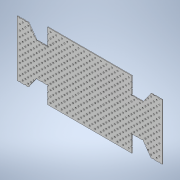
# Autodesk Inventor part: buildplate1
Saved by Autodesk Inventor 2020.1 (Build 241239000, 239)
## iProperties
Created: 2019-12-09
Part Number: buildplate1
Material: Aluminum 6061
Document SubType Name: Modeling
Designer: tbloo
Density: 2.7 g/cm^3
Appearance: Aluminum - Dark
Author: tbloo
Autodesk Inventor part; units mm, degrees
(part 1 of 2)
ref_plane "YZ Plane" through (0, 0, 0) normal (1, 0, 0) x (0, 1, 0)
ref_plane "XZ Plane" through (0, 0, 0) normal (0, 1, 0) x (-1, 0, 0)
ref_plane "XY Plane" through (0, 0, 0) normal (0, 0, 1) x (1, 0, 0)
sketch "Sketch1" plane through (0, 0, 0) normal (0, 0, 1) x (1, 0, 0)
  point P0 (0, 0)
sketch "Sketch2" plane through (0, 0, 0) normal (0, 0, 1) x (1, 0, 0)
  line L0 (32, 144) -> (-384, 144)
  line L1 (-384, 144) -> (-384, -48)
  line L2 (-384, -48) -> (32, -48)
  line L3 (32, -48) -> (32, 144)
  circle A0 centre (24, 128) radius 1.85
  circle A1 centre (16, 136) radius 1.85
  circle A2 centre (24, 112) radius 1.85
  circle A3 centre (16, 120) radius 1.85
  circle A4 centre (8, 128) radius 1.85
  circle A5 centre (0, 136) radius 1.85
  circle A6 centre (24, 112) radius 1.85
  circle A7 centre (16, 120) radius 1.85
  circle A8 centre (8, 112) radius 1.85
  circle A9 centre (16, 104) radius 1.85
  circle A10 centre (24, 96) radius 1.85
  circle A11 centre (16, 104) radius 1.85
  circle A12 centre (8, 96) radius 1.85
  circle A13 centre (16, 88) radius 1.85
  circle A14 centre (24, 80) radius 1.85
  circle A15 centre (16, 88) radius 1.85
  circle A16 centre (8, 80) radius 1.85
  circle A17 centre (16, 72) radius 1.85
  circle A18 centre (24, 64) radius 1.85
  circle A19 centre (16, 72) radius 1.85
  circle A20 centre (8, 64) radius 1.85
  circle A21 centre (16, 56) radius 1.85
  circle A22 centre (24, 48) radius 1.85
  circle A23 centre (16, 56) radius 1.85
  circle A24 centre (8, 48) radius 1.85
  circle A25 centre (16, 40) radius 1.85
  circle A26 centre (24, 32) radius 1.85
  circle A27 centre (16, 40) radius 1.85
  circle A28 centre (8, 32) radius 1.85
  circle A29 centre (16, 24) radius 1.85
  circle A30 centre (24, 16) radius 1.85
  circle A31 centre (16, 24) radius 1.85
  circle A32 centre (8, 16) radius 1.85
  circle A33 centre (16, 8) radius 1.85
  circle A34 centre (24, 0) radius 1.85
  circle A35 centre (16, 8) radius 1.85
  circle A36 centre (8, 0) radius 1.85
  circle A37 centre (16, -8) radius 1.85
  circle A38 centre (24, -16) radius 1.85
  circle A39 centre (16, -8) radius 1.85
  circle A40 centre (8, -16) radius 1.85
  circle A41 centre (16, -24) radius 1.85
  circle A42 centre (24, -32) radius 1.85
  circle A43 centre (16, -24) radius 1.85
  circle A44 centre (8, -32) radius 1.85
  circle A45 centre (16, -40) radius 1.85
  circle A46 centre (8, 128) radius 1.85
  circle A47 centre (0, 136) radius 1.85
  circle A48 centre (-8, 128) radius 1.85
  circle A49 centre (0, 120) radius 1.85
  circle A50 centre (8, 112) radius 1.85
  circle A51 centre (0, 120) radius 1.85
  circle A52 centre (-8, 112) radius 1.85
  circle A53 centre (0, 104) radius 1.85
  circle A54 centre (8, 96) radius 1.85
  circle A55 centre (0, 104) radius 1.85
  circle A56 centre (-8, 96) radius 1.85
  circle A57 centre (0, 88) radius 1.85
  circle A58 centre (8, 80) radius 1.85
  circle A59 centre (0, 88) radius 1.85
  circle A60 centre (-8, 80) radius 1.85
  circle A61 centre (0, 72) radius 1.85
  circle A62 centre (8, 64) radius 1.85
  circle A63 centre (0, 72) radius 1.85
  circle A64 centre (-8, 64) radius 1.85
  circle A65 centre (0, 56) radius 1.85
  circle A66 centre (8, 48) radius 1.85
  circle A67 centre (0, 56) radius 1.85
  circle A68 centre (-8, 48) radius 1.85
  circle A69 centre (0, 40) radius 1.85
  circle A70 centre (8, 32) radius 1.85
  circle A71 centre (0, 40) radius 1.85
  circle A72 centre (-8, 32) radius 1.85
  circle A73 centre (0, 24) radius 1.85
  circle A74 centre (8, 16) radius 1.85
  circle A75 centre (0, 24) radius 1.85
  circle A76 centre (-8, 16) radius 1.85
  circle A77 centre (0, 8) radius 1.85
  circle A78 centre (8, 0) radius 1.85
  circle A79 centre (0, 8) radius 1.85
  circle A80 centre (-8, 0) radius 1.85
  circle A81 centre (0, -8) radius 1.85
  circle A82 centre (8, -16) radius 1.85
  circle A83 centre (0, -8) radius 1.85
  circle A84 centre (-8, -16) radius 1.85
  circle A85 centre (0, -24) radius 1.85
  circle A86 centre (8, -32) radius 1.85
  circle A87 centre (0, -24) radius 1.85
  circle A88 centre (-8, -32) radius 1.85
  circle A89 centre (0, -40) radius 1.85
  circle A90 centre (-8, 128) radius 1.85
  circle A91 centre (-16, 136) radius 1.85
  circle A92 centre (-24, 128) radius 1.85
  circle A93 centre (-16, 120) radius 1.85
  circle A94 centre (-8, 112) radius 1.85
  circle A95 centre (-16, 120) radius 1.85
  circle A96 centre (-24, 112) radius 1.85
  circle A97 centre (-16, 104) radius 1.85
  circle A98 centre (-8, 96) radius 1.85
  circle A99 centre (-16, 104) radius 1.85
  circle A100 centre (-24, 96) radius 1.85
  circle A101 centre (-16, 88) radius 1.85
  circle A102 centre (-8, 80) radius 1.85
  circle A103 centre (-16, 88) radius 1.85
  circle A104 centre (-24, 80) radius 1.85
  circle A105 centre (-16, 72) radius 1.85
  circle A106 centre (-8, 64) radius 1.85
  circle A107 centre (-16, 72) radius 1.85
  circle A108 centre (-24, 64) radius 1.85
  circle A109 centre (-16, 56) radius 1.85
  circle A110 centre (-8, 48) radius 1.85
  circle A111 centre (-16, 56) radius 1.85
  circle A112 centre (-24, 48) radius 1.85
  circle A113 centre (-16, 40) radius 1.85
  circle A114 centre (-8, 32) radius 1.85
  circle A115 centre (-16, 40) radius 1.85
  circle A116 centre (-24, 32) radius 1.85
  circle A117 centre (-16, 24) radius 1.85
  circle A118 centre (-8, 16) radius 1.85
  circle A119 centre (-16, 24) radius 1.85
  circle A120 centre (-24, 16) radius 1.85
  circle A121 centre (-16, 8) radius 1.85
  circle A122 centre (-8, 0) radius 1.85
  circle A123 centre (-16, 8) radius 1.85
  circle A124 centre (-24, 0) radius 1.85
  circle A125 centre (-16, -8) radius 1.85
  circle A126 centre (-8, -16) radius 1.85
  circle A127 centre (-16, -8) radius 1.85
  circle A128 centre (-24, -16) radius 1.85
  circle A129 centre (-16, -24) radius 1.85
  circle A130 centre (-8, -32) radius 1.85
  circle A131 centre (-16, -24) radius 1.85
  circle A132 centre (-24, -32) radius 1.85
  circle A133 centre (-16, -40) radius 1.85
  circle A134 centre (-24, 128) radius 1.85
  circle A135 centre (-32, 136) radius 1.85
  circle A136 centre (-40, 128) radius 1.85
  circle A137 centre (-32, 120) radius 1.85
  circle A138 centre (-24, 112) radius 1.85
  circle A139 centre (-32, 120) radius 1.85
  circle A140 centre (-40, 112) radius 1.85
  circle A141 centre (-32, 104) radius 1.85
  circle A142 centre (-24, 96) radius 1.85
  circle A143 centre (-32, 104) radius 1.85
  circle A144 centre (-40, 96) radius 1.85
  circle A145 centre (-32, 88) radius 1.85
  circle A146 centre (-24, 80) radius 1.85
  circle A147 centre (-32, 88) radius 1.85
  circle A148 centre (-40, 80) radius 1.85
  circle A149 centre (-32, 72) radius 1.85
  circle A150 centre (-24, 64) radius 1.85
  circle A151 centre (-32, 72) radius 1.85
  circle A152 centre (-40, 64) radius 1.85
  circle A153 centre (-32, 56) radius 1.85
  circle A154 centre (-24, 48) radius 1.85
  circle A155 centre (-32, 56) radius 1.85
  circle A156 centre (-40, 48) radius 1.85
  circle A157 centre (-32, 40) radius 1.85
  circle A158 centre (-24, 32) radius 1.85
  circle A159 centre (-32, 40) radius 1.85
  circle A160 centre (-40, 32) radius 1.85
  circle A161 centre (-32, 24) radius 1.85
  circle A162 centre (-24, 16) radius 1.85
  circle A163 centre (-32, 24) radius 1.85
  circle A164 centre (-40, 16) radius 1.85
  circle A165 centre (-32, 8) radius 1.85
  circle A166 centre (-24, 0) radius 1.85
  circle A167 centre (-32, 8) radius 1.85
  circle A168 centre (-40, 0) radius 1.85
  circle A169 centre (-32, -8) radius 1.85
  circle A170 centre (-24, -16) radius 1.85
  circle A171 centre (-32, -8) radius 1.85
  circle A172 centre (-40, -16) radius 1.85
  circle A173 centre (-32, -24) radius 1.85
  circle A174 centre (-24, -32) radius 1.85
  circle A175 centre (-32, -24) radius 1.85
  circle A176 centre (-40, -32) radius 1.85
  circle A177 centre (-32, -40) radius 1.85
  circle A178 centre (-40, 128) radius 1.85
  circle A179 centre (-48, 136) radius 1.85
  circle A180 centre (-56, 128) radius 1.85
  circle A181 centre (-48, 120) radius 1.85
  circle A182 centre (-40, 112) radius 1.85
  circle A183 centre (-48, 120) radius 1.85
  circle A184 centre (-56, 112) radius 1.85
  circle A185 centre (-48, 104) radius 1.85
  circle A186 centre (-40, 96) radius 1.85
  circle A187 centre (-48, 104) radius 1.85
  circle A188 centre (-56, 96) radius 1.85
  circle A189 centre (-48, 88) radius 1.85
  circle A190 centre (-40, 80) radius 1.85
  circle A191 centre (-48, 88) radius 1.85
  circle A192 centre (-56, 80) radius 1.85
  circle A193 centre (-48, 72) radius 1.85
  circle A194 centre (-40, 64) radius 1.85
  circle A195 centre (-48, 72) radius 1.85
  circle A196 centre (-56, 64) radius 1.85
  circle A197 centre (-48, 56) radius 1.85
  circle A198 centre (-40, 48) radius 1.85
  circle A199 centre (-48, 56) radius 1.85
  circle A200 centre (-56, 48) radius 1.85
  circle A201 centre (-48, 40) radius 1.85
  circle A202 centre (-40, 32) radius 1.85
  circle A203 centre (-48, 40) radius 1.85
  circle A204 centre (-56, 32) radius 1.85
  circle A205 centre (-48, 24) radius 1.85
  circle A206 centre (-40, 16) radius 1.85
  circle A207 centre (-48, 24) radius 1.85
  circle A208 centre (-56, 16) radius 1.85
  circle A209 centre (-48, 8) radius 1.85
  circle A210 centre (-40, 0) radius 1.85
  circle A211 centre (-48, 8) radius 1.85
  circle A212 centre (-56, 0) radius 1.85
  circle A213 centre (-48, -8) radius 1.85
  circle A214 centre (-40, -16) radius 1.85
  circle A215 centre (-48, -8) radius 1.85
  circle A216 centre (-56, -16) radius 1.85
  circle A217 centre (-48, -24) radius 1.85
  circle A218 centre (-40, -32) radius 1.85
  circle A219 centre (-48, -24) radius 1.85
  circle A220 centre (-56, -32) radius 1.85
  circle A221 centre (-48, -40) radius 1.85
  circle A222 centre (-56, 128) radius 1.85
  circle A223 centre (-64, 136) radius 1.85
  circle A224 centre (-72, 128) radius 1.85
  circle A225 centre (-64, 120) radius 1.85
  circle A226 centre (-56, 112) radius 1.85
  circle A227 centre (-64, 120) radius 1.85
  circle A228 centre (-72, 112) radius 1.85
  circle A229 centre (-64, 104) radius 1.85
  circle A230 centre (-56, 96) radius 1.85
  circle A231 centre (-64, 104) radius 1.85
  circle A232 centre (-72, 96) radius 1.85
  circle A233 centre (-64, 88) radius 1.85
  circle A234 centre (-56, 80) radius 1.85
  circle A235 centre (-64, 88) radius 1.85
  circle A236 centre (-72, 80) radius 1.85
  circle A237 centre (-64, 72) radius 1.85
  circle A238 centre (-56, 64) radius 1.85
  circle A239 centre (-64, 72) radius 1.85
  circle A240 centre (-72, 64) radius 1.85
  circle A241 centre (-64, 56) radius 1.85
  circle A242 centre (-56, 48) radius 1.85
  circle A243 centre (-64, 56) radius 1.85
  circle A244 centre (-72, 48) radius 1.85
  circle A245 centre (-64, 40) radius 1.85
  circle A246 centre (-56, 32) radius 1.85
  circle A247 centre (-64, 40) radius 1.85
  circle A248 centre (-72, 32) radius 1.85
  circle A249 centre (-64, 24) radius 1.85
  circle A250 centre (-56, 16) radius 1.85
  circle A251 centre (-64, 24) radius 1.85
  circle A252 centre (-72, 16) radius 1.85
  circle A253 centre (-64, 8) radius 1.85
  circle A254 centre (-56, 0) radius 1.85
  circle A255 centre (-64, 8) radius 1.85
  circle A256 centre (-72, 0) radius 1.85
  circle A257 centre (-64, -8) radius 1.85
  circle A258 centre (-56, -16) radius 1.85
  circle A259 centre (-64, -8) radius 1.85
  circle A260 centre (-72, -16) radius 1.85
  circle A261 centre (-64, -24) radius 1.85
  circle A262 centre (-56, -32) radius 1.85
  circle A263 centre (-64, -24) radius 1.85
  circle A264 centre (-72, -32) radius 1.85
  circle A265 centre (-64, -40) radius 1.85
  circle A266 centre (-72, 128) radius 1.85
  circle A267 centre (-80, 136) radius 1.85
  circle A268 centre (-88, 128) radius 1.85
  circle A269 centre (-80, 120) radius 1.85
  circle A270 centre (-72, 112) radius 1.85
  circle A271 centre (-80, 120) radius 1.85
  circle A272 centre (-88, 112) radius 1.85
  circle A273 centre (-80, 104) radius 1.85
  circle A274 centre (-72, 96) radius 1.85
  circle A275 centre (-80, 104) radius 1.85
  circle A276 centre (-88, 96) radius 1.85
  circle A277 centre (-80, 88) radius 1.85
  circle A278 centre (-72, 80) radius 1.85
  circle A279 centre (-80, 88) radius 1.85
  circle A280 centre (-88, 80) radius 1.85
  circle A281 centre (-80, 72) radius 1.85
  circle A282 centre (-72, 64) radius 1.85
  circle A283 centre (-80, 72) radius 1.85
  circle A284 centre (-88, 64) radius 1.85
  circle A285 centre (-80, 56) radius 1.85
  circle A286 centre (-72, 48) radius 1.85
  circle A287 centre (-80, 56) radius 1.85
  circle A288 centre (-88, 48) radius 1.85
  circle A289 centre (-80, 40) radius 1.85
  circle A290 centre (-72, 32) radius 1.85
  circle A291 centre (-80, 40) radius 1.85
  circle A292 centre (-88, 32) radius 1.85
  circle A293 centre (-80, 24) radius 1.85
  circle A294 centre (-72, 16) radius 1.85
  circle A295 centre (-80, 24) radius 1.85
  circle A296 centre (-88, 16) radius 1.85
  circle A297 centre (-80, 8) radius 1.85
  circle A298 centre (-72, 0) radius 1.85
  circle A299 centre (-80, 8) radius 1.85
  circle A300 centre (-88, 0) radius 1.85
  circle A301 centre (-80, -8) radius 1.85
  circle A302 centre (-72, -16) radius 1.85
  circle A303 centre (-80, -8) radius 1.85
  circle A304 centre (-88, -16) radius 1.85
  circle A305 centre (-80, -24) radius 1.85
  circle A306 centre (-72, -32) radius 1.85
  circle A307 centre (-80, -24) radius 1.85
  circle A308 centre (-88, -32) radius 1.85
  circle A309 centre (-80, -40) radius 1.85
  circle A310 centre (-88, 128) radius 1.85
  circle A311 centre (-96, 136) radius 1.85
  circle A312 centre (-104, 128) radius 1.85
  circle A313 centre (-96, 120) radius 1.85
  circle A314 centre (-88, 112) radius 1.85
  circle A315 centre (-96, 120) radius 1.85
  circle A316 centre (-104, 112) radius 1.85
  circle A317 centre (-96, 104) radius 1.85
  circle A318 centre (-88, 96) radius 1.85
  circle A319 centre (-96, 104) radius 1.85
  circle A320 centre (-104, 96) radius 1.85
  circle A321 centre (-96, 88) radius 1.85
  circle A322 centre (-88, 80) radius 1.85
  circle A323 centre (-96, 88) radius 1.85
  circle A324 centre (-104, 80) radius 1.85
  circle A325 centre (-96, 72) radius 1.85
  circle A326 centre (-88, 64) radius 1.85
  circle A327 centre (-96, 72) radius 1.85
  circle A328 centre (-104, 64) radius 1.85
  circle A329 centre (-96, 56) radius 1.85
  circle A330 centre (-88, 48) radius 1.85
  circle A331 centre (-96, 56) radius 1.85
  circle A332 centre (-104, 48) radius 1.85
  circle A333 centre (-96, 40) radius 1.85
  circle A334 centre (-88, 32) radius 1.85
  circle A335 centre (-96, 40) radius 1.85
  circle A336 centre (-104, 32) radius 1.85
  circle A337 centre (-96, 24) radius 1.85
  circle A338 centre (-88, 16) radius 1.85
  circle A339 centre (-96, 24) radius 1.85
  circle A340 centre (-104, 16) radius 1.85
  circle A341 centre (-96, 8) radius 1.85
  circle A342 centre (-88, 0) radius 1.85
  circle A343 centre (-96, 8) radius 1.85
  circle A344 centre (-104, 0) radius 1.85
  circle A345 centre (-96, -8) radius 1.85
  circle A346 centre (-88, -16) radius 1.85
  circle A347 centre (-96, -8) radius 1.85
  circle A348 centre (-104, -16) radius 1.85
  circle A349 centre (-96, -24) radius 1.85
  circle A350 centre (-88, -32) radius 1.85
  circle A351 centre (-96, -24) radius 1.85
  circle A352 centre (-104, -32) radius 1.85
  circle A353 centre (-96, -40) radius 1.85
  circle A354 centre (-104, 128) radius 1.85
  circle A355 centre (-112, 136) radius 1.85
  circle A356 centre (-120, 128) radius 1.85
  circle A357 centre (-112, 120) radius 1.85
  circle A358 centre (-104, 112) radius 1.85
  circle A359 centre (-112, 120) radius 1.85
  circle A360 centre (-120, 112) radius 1.85
  circle A361 centre (-112, 104) radius 1.85
  circle A362 centre (-104, 96) radius 1.85
  circle A363 centre (-112, 104) radius 1.85
  circle A364 centre (-120, 96) radius 1.85
  circle A365 centre (-112, 88) radius 1.85
  circle A366 centre (-104, 80) radius 1.85
  circle A367 centre (-112, 88) radius 1.85
  circle A368 centre (-120, 80) radius 1.85
  circle A369 centre (-112, 72) radius 1.85
  circle A370 centre (-104, 64) radius 1.85
  circle A371 centre (-112, 72) radius 1.85
  circle A372 centre (-120, 64) radius 1.85
  circle A373 centre (-112, 56) radius 1.85
  circle A374 centre (-104, 48) radius 1.85
  circle A375 centre (-112, 56) radius 1.85
  circle A376 centre (-120, 48) radius 1.85
  circle A377 centre (-112, 40) radius 1.85
  circle A378 centre (-104, 32) radius 1.85
  circle A379 centre (-112, 40) radius 1.85
  circle A380 centre (-120, 32) radius 1.85
  circle A381 centre (-112, 24) radius 1.85
  circle A382 centre (-104, 16) radius 1.85
  circle A383 centre (-112, 24) radius 1.85
  circle A384 centre (-120, 16) radius 1.85
  circle A385 centre (-112, 8) radius 1.85
  circle A386 centre (-104, 0) radius 1.85
  circle A387 centre (-112, 8) radius 1.85
  circle A388 centre (-120, 0) radius 1.85
  circle A389 centre (-112, -8) radius 1.85
  circle A390 centre (-104, -16) radius 1.85
  circle A391 centre (-112, -8) radius 1.85
  circle A392 centre (-120, -16) radius 1.85
  circle A393 centre (-112, -24) radius 1.85
  circle A394 centre (-104, -32) radius 1.85
  circle A395 centre (-112, -24) radius 1.85
  circle A396 centre (-120, -32) radius 1.85
  circle A397 centre (-112, -40) radius 1.85
  circle A398 centre (-120, 128) radius 1.85
  circle A399 centre (-128, 136) radius 1.85
  circle A400 centre (-136, 128) radius 1.85
  circle A401 centre (-128, 120) radius 1.85
  circle A402 centre (-120, 112) radius 1.85
  circle A403 centre (-128, 120) radius 1.85
  circle A404 centre (-136, 112) radius 1.85
  circle A405 centre (-128, 104) radius 1.85
  circle A406 centre (-120, 96) radius 1.85
  circle A407 centre (-128, 104) radius 1.85
  circle A408 centre (-136, 96) radius 1.85
  circle A409 centre (-128, 88) radius 1.85
  circle A410 centre (-120, 80) radius 1.85
  circle A411 centre (-128, 88) radius 1.85
  circle A412 centre (-136, 80) radius 1.85
  circle A413 centre (-128, 72) radius 1.85
  circle A414 centre (-120, 64) radius 1.85
  circle A415 centre (-128, 72) radius 1.85
  circle A416 centre (-136, 64) radius 1.85
  circle A417 centre (-128, 56) radius 1.85
  circle A418 centre (-120, 48) radius 1.85
  circle A419 centre (-128, 56) radius 1.85
  circle A420 centre (-136, 48) radius 1.85
  circle A421 centre (-128, 40) radius 1.85
  circle A422 centre (-120, 32) radius 1.85
  circle A423 centre (-128, 40) radius 1.85
  circle A424 centre (-136, 32) radius 1.85
  circle A425 centre (-128, 24) radius 1.85
  circle A426 centre (-120, 16) radius 1.85
  circle A427 centre (-128, 24) radius 1.85
  circle A428 centre (-136, 16) radius 1.85
  circle A429 centre (-128, 8) radius 1.85
  circle A430 centre (-120, 0) radius 1.85
  circle A431 centre (-128, 8) radius 1.85
  circle A432 centre (-136, 0) radius 1.85
  circle A433 centre (-128, -8) radius 1.85
  circle A434 centre (-120, -16) radius 1.85
  circle A435 centre (-128, -8) radius 1.85
  circle A436 centre (-136, -16) radius 1.85
  circle A437 centre (-128, -24) radius 1.85
  circle A438 centre (-120, -32) radius 1.85
  circle A439 centre (-128, -24) radius 1.85
  circle A440 centre (-136, -32) radius 1.85
  circle A441 centre (-128, -40) radius 1.85
  circle A442 centre (-136, 128) radius 1.85
  circle A443 centre (-144, 136) radius 1.85
  circle A444 centre (-152, 128) radius 1.85
  circle A445 centre (-144, 120) radius 1.85
  circle A446 centre (-136, 112) radius 1.85
  circle A447 centre (-144, 120) radius 1.85
  circle A448 centre (-152, 112) radius 1.85
  circle A449 centre (-144, 104) radius 1.85
  circle A450 centre (-136, 96) radius 1.85
  circle A451 centre (-144, 104) radius 1.85
  circle A452 centre (-152, 96) radius 1.85
  circle A453 centre (-144, 88) radius 1.85
  circle A454 centre (-136, 80) radius 1.85
  circle A455 centre (-144, 88) radius 1.85
  circle A456 centre (-152, 80) radius 1.85
  circle A457 centre (-144, 72) radius 1.85
  circle A458 centre (-136, 64) radius 1.85
  circle A459 centre (-144, 72) radius 1.85
  circle A460 centre (-152, 64) radius 1.85
  circle A461 centre (-144, 56) radius 1.85
  circle A462 centre (-136, 48) radius 1.85
  circle A463 centre (-144, 56) radius 1.85
  circle A464 centre (-152, 48) radius 1.85
  circle A465 centre (-144, 40) radius 1.85
  circle A466 centre (-136, 32) radius 1.85
  circle A467 centre (-144, 40) radius 1.85
  circle A468 centre (-152, 32) radius 1.85
  circle A469 centre (-144, 24) radius 1.85
  circle A470 centre (-136, 16) radius 1.85
  circle A471 centre (-144, 24) radius 1.85
  circle A472 centre (-152, 16) radius 1.85
  circle A473 centre (-144, 8) radius 1.85
  circle A474 centre (-136, 0) radius 1.85
  circle A475 centre (-144, 8) radius 1.85
  circle A476 centre (-152, 0) radius 1.85
  circle A477 centre (-144, -8) radius 1.85
  circle A478 centre (-136, -16) radius 1.85
  circle A479 centre (-144, -8) radius 1.85
  circle A480 centre (-152, -16) radius 1.85
  circle A481 centre (-144, -24) radius 1.85
  circle A482 centre (-136, -32) radius 1.85
  circle A483 centre (-144, -24) radius 1.85
  circle A484 centre (-152, -32) radius 1.85
  circle A485 centre (-144, -40) radius 1.85
  circle A486 centre (-152, 128) radius 1.85
  circle A487 centre (-160, 136) radius 1.85
  circle A488 centre (-168, 128) radius 1.85
  circle A489 centre (-160, 120) radius 1.85
  circle A490 centre (-152, 112) radius 1.85
  circle A491 centre (-160, 120) radius 1.85
  circle A492 centre (-168, 112) radius 1.85
  circle A493 centre (-160, 104) radius 1.85
  circle A494 centre (-152, 96) radius 1.85
  circle A495 centre (-160, 104) radius 1.85
  circle A496 centre (-168, 96) radius 1.85
  circle A497 centre (-160, 88) radius 1.85
  circle A498 centre (-152, 80) radius 1.85
  circle A499 centre (-160, 88) radius 1.85
  circle A500 centre (-168, 80) radius 1.85
  circle A501 centre (-160, 72) radius 1.85
  circle A502 centre (-152, 64) radius 1.85
  circle A503 centre (-160, 72) radius 1.85
  circle A504 centre (-168, 64) radius 1.85
  circle A505 centre (-160, 56) radius 1.85
  circle A506 centre (-152, 48) radius 1.85
  circle A507 centre (-160, 56) radius 1.85
  circle A508 centre (-168, 48) radius 1.85
  circle A509 centre (-160, 40) radius 1.85
  circle A510 centre (-152, 32) radius 1.85
  circle A511 centre (-160, 40) radius 1.85
  circle A512 centre (-168, 32) radius 1.85
  circle A513 centre (-160, 24) radius 1.85
  circle A514 centre (-152, 16) radius 1.85
  circle A515 centre (-160, 24) radius 1.85
  circle A516 centre (-168, 16) radius 1.85
  circle A517 centre (-160, 8) radius 1.85
  circle A518 centre (-152, 0) radius 1.85
  circle A519 centre (-160, 8) radius 1.85
  circle A520 centre (-168, 0) radius 1.85
  circle A521 centre (-160, -8) radius 1.85
  circle A522 centre (-152, -16) radius 1.85
  circle A523 centre (-160, -8) radius 1.85
  circle A524 centre (-168, -16) radius 1.85
  circle A525 centre (-160, -24) radius 1.85
  circle A526 centre (-152, -32) radius 1.85
  circle A527 centre (-160, -24) radius 1.85
  circle A528 centre (-168, -32) radius 1.85
  circle A529 centre (-160, -40) radius 1.85
  circle A530 centre (-168, 128) radius 1.85
  circle A531 centre (-176, 136) radius 1.85
  circle A532 centre (-184, 128) radius 1.85
  circle A533 centre (-176, 120) radius 1.85
  circle A534 centre (-168, 112) radius 1.85
  circle A535 centre (-176, 120) radius 1.85
  circle A536 centre (-184, 112) radius 1.85
  circle A537 centre (-176, 104) radius 1.85
  circle A538 centre (-168, 96) radius 1.85
  circle A539 centre (-176, 104) radius 1.85
  circle A540 centre (-184, 96) radius 1.85
  circle A541 centre (-176, 88) radius 1.85
  circle A542 centre (-168, 80) radius 1.85
  circle A543 centre (-176, 88) radius 1.85
  circle A544 centre (-184, 80) radius 1.85
  circle A545 centre (-176, 72) radius 1.85
  circle A546 centre (-168, 64) radius 1.85
  circle A547 centre (-176, 72) radius 1.85
  circle A548 centre (-184, 64) radius 1.85
  circle A549 centre (-176, 56) radius 1.85
  circle A550 centre (-168, 48) radius 1.85
  circle A551 centre (-176, 56) radius 1.85
  circle A552 centre (-184, 48) radius 1.85
  circle A553 centre (-176, 40) radius 1.85
  circle A554 centre (-168, 32) radius 1.85
  circle A555 centre (-176, 40) radius 1.85
  circle A556 centre (-184, 32) radius 1.85
  circle A557 centre (-176, 24) radius 1.85
  circle A558 centre (-168, 16) radius 1.85
  circle A559 centre (-176, 24) radius 1.85
  circle A560 centre (-184, 16) radius 1.85
  circle A561 centre (-176, 8) radius 1.85
  circle A562 centre (-168, 0) radius 1.85
  circle A563 centre (-176, 8) radius 1.85
  circle A564 centre (-184, 0) radius 1.85
  circle A565 centre (-176, -8) radius 1.85
  circle A566 centre (-168, -16) radius 1.85
  circle A567 centre (-176, -8) radius 1.85
  circle A568 centre (-184, -16) radius 1.85
  circle A569 centre (-176, -24) radius 1.85
  circle A570 centre (-168, -32) radius 1.85
  circle A571 centre (-176, -24) radius 1.85
  circle A572 centre (-184, -32) radius 1.85
  circle A573 centre (-176, -40) radius 1.85
  circle A574 centre (-184, 128) radius 1.85
  circle A575 centre (-192, 136) radius 1.85
  circle A576 centre (-200, 128) radius 1.85
  circle A577 centre (-192, 120) radius 1.85
  circle A578 centre (-184, 112) radius 1.85
  circle A579 centre (-192, 120) radius 1.85
  circle A580 centre (-200, 112) radius 1.85
  circle A581 centre (-192, 104) radius 1.85
  circle A582 centre (-184, 96) radius 1.85
  circle A583 centre (-192, 104) radius 1.85
  circle A584 centre (-200, 96) radius 1.85
  circle A585 centre (-192, 88) radius 1.85
  circle A586 centre (-184, 80) radius 1.85
  circle A587 centre (-192, 88) radius 1.85
  circle A588 centre (-200, 80) radius 1.85
  circle A589 centre (-192, 72) radius 1.85
  circle A590 centre (-184, 64) radius 1.85
  circle A591 centre (-192, 72) radius 1.85
  circle A592 centre (-200, 64) radius 1.85
  circle A593 centre (-192, 56) radius 1.85
  circle A594 centre (-184, 48) radius 1.85
  circle A595 centre (-192, 56) radius 1.85
  circle A596 centre (-200, 48) radius 1.85
  circle A597 centre (-192, 40) radius 1.85
  circle A598 centre (-184, 32) radius 1.85
  circle A599 centre (-192, 40) radius 1.85
  circle A600 centre (-200, 32) radius 1.85
  circle A601 centre (-192, 24) radius 1.85
  circle A602 centre (-184, 16) radius 1.85
  circle A603 centre (-192, 24) radius 1.85
  circle A604 centre (-200, 16) radius 1.85
  circle A605 centre (-192, 8) radius 1.85
  circle A606 centre (-184, 0) radius 1.85
  circle A607 centre (-192, 8) radius 1.85
  circle A608 centre (-200, 0) radius 1.85
  circle A609 centre (-192, -8) radius 1.85
  circle A610 centre (-184, -16) radius 1.85
  circle A611 centre (-192, -8) radius 1.85
  circle A612 centre (-200, -16) radius 1.85
  circle A613 centre (-192, -24) radius 1.85
  circle A614 centre (-184, -32) radius 1.85
  circle A615 centre (-192, -24) radius 1.85
  circle A616 centre (-200, -32) radius 1.85
  circle A617 centre (-192, -40) radius 1.85
  circle A618 centre (-200, 128) radius 1.85
  circle A619 centre (-208, 136) radius 1.85
  circle A620 centre (-216, 128) radius 1.85
  circle A621 centre (-208, 120) radius 1.85
  circle A622 centre (-200, 112) radius 1.85
  circle A623 centre (-208, 120) radius 1.85
  circle A624 centre (-216, 112) radius 1.85
  circle A625 centre (-208, 104) radius 1.85
  circle A626 centre (-200, 96) radius 1.85
  circle A627 centre (-208, 104) radius 1.85
  circle A628 centre (-216, 96) radius 1.85
  circle A629 centre (-208, 88) radius 1.85
  circle A630 centre (-200, 80) radius 1.85
  circle A631 centre (-208, 88) radius 1.85
  circle A632 centre (-216, 80) radius 1.85
  circle A633 centre (-208, 72) radius 1.85
  circle A634 centre (-200, 64) radius 1.85
  circle A635 centre (-208, 72) radius 1.85
  circle A636 centre (-216, 64) radius 1.85
  circle A637 centre (-208, 56) radius 1.85
  circle A638 centre (-200, 48) radius 1.85
  circle A639 centre (-208, 56) radius 1.85
  circle A640 centre (-216, 48) radius 1.85
  circle A641 centre (-208, 40) radius 1.85
  circle A642 centre (-200, 32) radius 1.85
  circle A643 centre (-208, 40) radius 1.85
  circle A644 centre (-216, 32) radius 1.85
  circle A645 centre (-208, 24) radius 1.85
  circle A646 centre (-200, 16) radius 1.85
  circle A647 centre (-208, 24) radius 1.85
  circle A648 centre (-216, 16) radius 1.85
  circle A649 centre (-208, 8) radius 1.85
  circle A650 centre (-200, 0) radius 1.85
  circle A651 centre (-208, 8) radius 1.85
  circle A652 centre (-216, 0) radius 1.85
  circle A653 centre (-208, -8) radius 1.85
  circle A654 centre (-200, -16) radius 1.85
  circle A655 centre (-208, -8) radius 1.85
  circle A656 centre (-216, -16) radius 1.85
  circle A657 centre (-208, -24) radius 1.85
  circle A658 centre (-200, -32) radius 1.85
  circle A659 centre (-208, -24) radius 1.85
  circle A660 centre (-216, -32) radius 1.85
  circle A661 centre (-208, -40) radius 1.85
  circle A662 centre (-216, 128) radius 1.85
  circle A663 centre (-224, 136) radius 1.85
  circle A664 centre (-232, 128) radius 1.85
  circle A665 centre (-224, 120) radius 1.85
  circle A666 centre (-216, 112) radius 1.85
  circle A667 centre (-224, 120) radius 1.85
  circle A668 centre (-232, 112) radius 1.85
  circle A669 centre (-224, 104) radius 1.85
  circle A670 centre (-216, 96) radius 1.85
  circle A671 centre (-224, 104) radius 1.85
  circle A672 centre (-232, 96) radius 1.85
  circle A673 centre (-224, 88) radius 1.85
  circle A674 centre (-216, 80) radius 1.85
  circle A675 centre (-224, 88) radius 1.85
  circle A676 centre (-232, 80) radius 1.85
  circle A677 centre (-224, 72) radius 1.85
  circle A678 centre (-216, 64) radius 1.85
  circle A679 centre (-224, 72) radius 1.85
  circle A680 centre (-232, 64) radius 1.85
  circle A681 centre (-224, 56) radius 1.85
  circle A682 centre (-216, 48) radius 1.85
  circle A683 centre (-224, 56) radius 1.85
  circle A684 centre (-232, 48) radius 1.85
  circle A685 centre (-224, 40) radius 1.85
  circle A686 centre (-216, 32) radius 1.85
  circle A687 centre (-224, 40) radius 1.85
  circle A688 centre (-232, 32) radius 1.85
  circle A689 centre (-224, 24) radius 1.85
  circle A690 centre (-216, 16) radius 1.85
  circle A691 centre (-224, 24) radius 1.85
  circle A692 centre (-232, 16) radius 1.85
  circle A693 centre (-224, 8) radius 1.85
  circle A694 centre (-216, 0) radius 1.85
  circle A695 centre (-224, 8) radius 1.85
  circle A696 centre (-232, 0) radius 1.85
  circle A697 centre (-224, -8) radius 1.85
  circle A698 centre (-216, -16) radius 1.85
  circle A699 centre (-224, -8) radius 1.85
  circle A700 centre (-232, -16) radius 1.85
  circle A701 centre (-224, -24) radius 1.85
  circle A702 centre (-216, -32) radius 1.85
  circle A703 centre (-224, -24) radius 1.85
  circle A704 centre (-232, -32) radius 1.85
  circle A705 centre (-224, -40) radius 1.85
  circle A706 centre (-232, 128) radius 1.85
  circle A707 centre (-240, 136) radius 1.85
  circle A708 centre (-248, 128) radius 1.85
  circle A709 centre (-240, 120) radius 1.85
  circle A710 centre (-232, 112) radius 1.85
  circle A711 centre (-240, 120) radius 1.85
  circle A712 centre (-248, 112) radius 1.85
  circle A713 centre (-240, 104) radius 1.85
  circle A714 centre (-232, 96) radius 1.85
  circle A715 centre (-240, 104) radius 1.85
  circle A716 centre (-248, 96) radius 1.85
  circle A717 centre (-240, 88) radius 1.85
  circle A718 centre (-232, 80) radius 1.85
  circle A719 centre (-240, 88) radius 1.85
  circle A720 centre (-248, 80) radius 1.85
  circle A721 centre (-240, 72) radius 1.85
  circle A722 centre (-232, 64) radius 1.85
  circle A723 centre (-240, 72) radius 1.85
  circle A724 centre (-248, 64) radius 1.85
  circle A725 centre (-240, 56) radius 1.85
  circle A726 centre (-232, 48) radius 1.85
  circle A727 centre (-240, 56) radius 1.85
  circle A728 centre (-248, 48) radius 1.85
  circle A729 centre (-240, 40) radius 1.85
  circle A730 centre (-232, 32) radius 1.85
  circle A731 centre (-240, 40) radius 1.85
  circle A732 centre (-248, 32) radius 1.85
  circle A733 centre (-240, 24) radius 1.85
  circle A734 centre (-232, 16) radius 1.85
  circle A735 centre (-240, 24) radius 1.85
  circle A736 centre (-248, 16) radius 1.85
  circle A737 centre (-240, 8) radius 1.85
  circle A738 centre (-232, 0) radius 1.85
  circle A739 centre (-240, 8) radius 1.85
  circle A740 centre (-248, 0) radius 1.85
  circle A741 centre (-240, -8) radius 1.85
  circle A742 centre (-232, -16) radius 1.85
  circle A743 centre (-240, -8) radius 1.85
  circle A744 centre (-248, -16) radius 1.85
  circle A745 centre (-240, -24) radius 1.85
  circle A746 centre (-232, -32) radius 1.85
  circle A747 centre (-240, -24) radius 1.85
  circle A748 centre (-248, -32) radius 1.85
  circle A749 centre (-240, -40) radius 1.85
  circle A750 centre (-248, 128) radius 1.85
  circle A751 centre (-256, 136) radius 1.85
  circle A752 centre (-264, 128) radius 1.85
  circle A753 centre (-256, 120) radius 1.85
  circle A754 centre (-248, 112) radius 1.85
  circle A755 centre (-256, 120) radius 1.85
  circle A756 centre (-264, 112) radius 1.85
  circle A757 centre (-256, 104) radius 1.85
  circle A758 centre (-248, 96) radius 1.85
  circle A759 centre (-256, 104) radius 1.85
  circle A760 centre (-264, 96) radius 1.85
  circle A761 centre (-256, 88) radius 1.85
  circle A762 centre (-248, 80) radius 1.85
  circle A763 centre (-256, 88) radius 1.85
  circle A764 centre (-264, 80) radius 1.85
  circle A765 centre (-256, 72) radius 1.85
  circle A766 centre (-248, 64) radius 1.85
  circle A767 centre (-256, 72) radius 1.85
  circle A768 centre (-264, 64) radius 1.85
  circle A769 centre (-256, 56) radius 1.85
  circle A770 centre (-248, 48) radius 1.85
  circle A771 centre (-256, 56) radius 1.85
  circle A772 centre (-264, 48) radius 1.85
  circle A773 centre (-256, 40) radius 1.85
  circle A774 centre (-248, 32) radius 1.85
  circle A775 centre (-256, 40) radius 1.85
  circle A776 centre (-264, 32) radius 1.85
  circle A777 centre (-256, 24) radius 1.85
  circle A778 centre (-248, 16) radius 1.85
  circle A779 centre (-256, 24) radius 1.85
  circle A780 centre (-264, 16) radius 1.85
  circle A781 centre (-256, 8) radius 1.85
  circle A782 centre (-248, 0) radius 1.85
  circle A783 centre (-256, 8) radius 1.85
  circle A784 centre (-264, 0) radius 1.85
  circle A785 centre (-256, -8) radius 1.85
  circle A786 centre (-248, -16) radius 1.85
  circle A787 centre (-256, -8) radius 1.85
  circle A788 centre (-264, -16) radius 1.85
  circle A789 centre (-256, -24) radius 1.85
  circle A790 centre (-248, -32) radius 1.85
  circle A791 centre (-256, -24) radius 1.85
  circle A792 centre (-264, -32) radius 1.85
  circle A793 centre (-256, -40) radius 1.85
  circle A794 centre (-264, 128) radius 1.85
  circle A795 centre (-272, 136) radius 1.85
  circle A796 centre (-280, 128) radius 1.85
  circle A797 centre (-272, 120) radius 1.85
  circle A798 centre (-264, 112) radius 1.85
  circle A799 centre (-272, 120) radius 1.85
  circle A800 centre (-280, 112) radius 1.85
  circle A801 centre (-272, 104) radius 1.85
  circle A802 centre (-264, 96) radius 1.85
  circle A803 centre (-272, 104) radius 1.85
  circle A804 centre (-280, 96) radius 1.85
  circle A805 centre (-272, 88) radius 1.85
  circle A806 centre (-264, 80) radius 1.85
  circle A807 centre (-272, 88) radius 1.85
  circle A808 centre (-280, 80) radius 1.85
  circle A809 centre (-272, 72) radius 1.85
  circle A810 centre (-264, 64) radius 1.85
  circle A811 centre (-272, 72) radius 1.85
  circle A812 centre (-280, 64) radius 1.85
  circle A813 centre (-272, 56) radius 1.85
  circle A814 centre (-264, 48) radius 1.85
  circle A815 centre (-272, 56) radius 1.85
  circle A816 centre (-280, 48) radius 1.85
  circle A817 centre (-272, 40) radius 1.85
  circle A818 centre (-264, 32) radius 1.85
  circle A819 centre (-272, 40) radius 1.85
  circle A820 centre (-280, 32) radius 1.85
  circle A821 centre (-272, 24) radius 1.85
  circle A822 centre (-264, 16) radius 1.85
  circle A823 centre (-272, 24) radius 1.85
  circle A824 centre (-280, 16) radius 1.85
  circle A825 centre (-272, 8) radius 1.85
  circle A826 centre (-264, 0) radius 1.85
  circle A827 centre (-272, 8) radius 1.85
  circle A828 centre (-280, 0) radius 1.85
  circle A829 centre (-272, -8) radius 1.85
  circle A830 centre (-264, -16) radius 1.85
  circle A831 centre (-272, -8) radius 1.85
  circle A832 centre (-280, -16) radius 1.85
  circle A833 centre (-272, -24) radius 1.85
  circle A834 centre (-264, -32) radius 1.85
  circle A835 centre (-272, -24) radius 1.85
  circle A836 centre (-280, -32) radius 1.85
  circle A837 centre (-272, -40) radius 1.85
  circle A838 centre (-280, 128) radius 1.85
  circle A839 centre (-288, 136) radius 1.85
  circle A840 centre (-296, 128) radius 1.85
  circle A841 centre (-288, 120) radius 1.85
  circle A842 centre (-280, 112) radius 1.85
  circle A843 centre (-288, 120) radius 1.85
  circle A844 centre (-296, 112) radius 1.85
  circle A845 centre (-288, 104) radius 1.85
  circle A846 centre (-280, 96) radius 1.85
  circle A847 centre (-288, 104) radius 1.85
  circle A848 centre (-296, 96) radius 1.85
  circle A849 centre (-288, 88) radius 1.85
  circle A850 centre (-280, 80) radius 1.85
  circle A851 centre (-288, 88) radius 1.85
  circle A852 centre (-296, 80) radius 1.85
  circle A853 centre (-288, 72) radius 1.85
  circle A854 centre (-280, 64) radius 1.85
  circle A855 centre (-288, 72) radius 1.85
  circle A856 centre (-296, 64) radius 1.85
  circle A857 centre (-288, 56) radius 1.85
  circle A858 centre (-280, 48) radius 1.85
  circle A859 centre (-288, 56) radius 1.85
  circle A860 centre (-296, 48) radius 1.85
  circle A861 centre (-288, 40) radius 1.85
  circle A862 centre (-280, 32) radius 1.85
  circle A863 centre (-288, 40) radius 1.85
  circle A864 centre (-296, 32) radius 1.85
  circle A865 centre (-288, 24) radius 1.85
  circle A866 centre (-280, 16) radius 1.85
  circle A867 centre (-288, 24) radius 1.85
  circle A868 centre (-296, 16) radius 1.85
  circle A869 centre (-288, 8) radius 1.85
  circle A870 centre (-280, 0) radius 1.85
  circle A871 centre (-288, 8) radius 1.85
  circle A872 centre (-296, 0) radius 1.85
  circle A873 centre (-288, -8) radius 1.85
  circle A874 centre (-280, -16) radius 1.85
  circle A875 centre (-288, -8) radius 1.85
  circle A876 centre (-296, -16) radius 1.85
  circle A877 centre (-288, -24) radius 1.85
  circle A878 centre (-280, -32) radius 1.85
  circle A879 centre (-288, -24) radius 1.85
  circle A880 centre (-296, -32) radius 1.85
  circle A881 centre (-288, -40) radius 1.85
  circle A882 centre (-296, 128) radius 1.85
  circle A883 centre (-304, 136) radius 1.85
  circle A884 centre (-312, 128) radius 1.85
  circle A885 centre (-304, 120) radius 1.85
  circle A886 centre (-296, 112) radius 1.85
  circle A887 centre (-304, 120) radius 1.85
  circle A888 centre (-312, 112) radius 1.85
  circle A889 centre (-304, 104) radius 1.85
  circle A890 centre (-296, 96) radius 1.85
  circle A891 centre (-304, 104) radius 1.85
  circle A892 centre (-312, 96) radius 1.85
  circle A893 centre (-304, 88) radius 1.85
  circle A894 centre (-296, 80) radius 1.85
  circle A895 centre (-304, 88) radius 1.85
  circle A896 centre (-312, 80) radius 1.85
  circle A897 centre (-304, 72) radius 1.85
  circle A898 centre (-296, 64) radius 1.85
  circle A899 centre (-304, 72) radius 1.85
  circle A900 centre (-312, 64) radius 1.85
  circle A901 centre (-304, 56) radius 1.85
  circle A902 centre (-296, 48) radius 1.85
  circle A903 centre (-304, 56) radius 1.85
  circle A904 centre (-312, 48) radius 1.85
  circle A905 centre (-304, 40) radius 1.85
  circle A906 centre (-296, 32) radius 1.85
  circle A907 centre (-304, 40) radius 1.85
  circle A908 centre (-312, 32) radius 1.85
  circle A909 centre (-304, 24) radius 1.85
  circle A910 centre (-296, 16) radius 1.85
  circle A911 centre (-304, 24) radius 1.85
  circle A912 centre (-312, 16) radius 1.85
  circle A913 centre (-304, 8) radius 1.85
  circle A914 centre (-296, 0) radius 1.85
  circle A915 centre (-304, 8) radius 1.85
  circle A916 centre (-312, 0) radius 1.85
  circle A917 centre (-304, -8) radius 1.85
  circle A918 centre (-296, -16) radius 1.85
  circle A919 centre (-304, -8) radius 1.85
  circle A920 centre (-312, -16) radius 1.85
  circle A921 centre (-304, -24) radius 1.85
  circle A922 centre (-296, -32) radius 1.85
  circle A923 centre (-304, -24) radius 1.85
  circle A924 centre (-312, -32) radius 1.85
  circle A925 centre (-304, -40) radius 1.85
  circle A926 centre (-312, 128) radius 1.85
  circle A927 centre (-320, 136) radius 1.85
  circle A928 centre (-328, 128) radius 1.85
  circle A929 centre (-320, 120) radius 1.85
  circle A930 centre (-312, 112) radius 1.85
  circle A931 centre (-320, 120) radius 1.85
  circle A932 centre (-328, 112) radius 1.85
  circle A933 centre (-320, 104) radius 1.85
  circle A934 centre (-312, 96) radius 1.85
  circle A935 centre (-320, 104) radius 1.85
  circle A936 centre (-328, 96) radius 1.85
  circle A937 centre (-320, 88) radius 1.85
  circle A938 centre (-312, 80) radius 1.85
  circle A939 centre (-320, 88) radius 1.85
  circle A940 centre (-328, 80) radius 1.85
  circle A941 centre (-320, 72) radius 1.85
  circle A942 centre (-312, 64) radius 1.85
  circle A943 centre (-320, 72) radius 1.85
  circle A944 centre (-328, 64) radius 1.85
  circle A945 centre (-320, 56) radius 1.85
  circle A946 centre (-312, 48) radius 1.85
  circle A947 centre (-320, 56) radius 1.85
  circle A948 centre (-328, 48) radius 1.85
  circle A949 centre (-320, 40) radius 1.85
  circle A950 centre (-312, 32) radius 1.85
  circle A951 centre (-320, 40) radius 1.85
  circle A952 centre (-328, 32) radius 1.85
  circle A953 centre (-320, 24) radius 1.85
  circle A954 centre (-312, 16) radius 1.85
  circle A955 centre (-320, 24) radius 1.85
  circle A956 centre (-328, 16) radius 1.85
  circle A957 centre (-320, 8) radius 1.85
  circle A958 centre (-312, 0) radius 1.85
  circle A959 centre (-320, 8) radius 1.85
  circle A960 centre (-328, 0) radius 1.85
  circle A961 centre (-320, -8) radius 1.85
  circle A962 centre (-312, -16) radius 1.85
  circle A963 centre (-320, -8) radius 1.85
  circle A964 centre (-328, -16) radius 1.85
  circle A965 centre (-320, -24) radius 1.85
  circle A966 centre (-312, -32) radius 1.85
  circle A967 centre (-320, -24) radius 1.85
  circle A968 centre (-328, -32) radius 1.85
  circle A969 centre (-320, -40) radius 1.85
  circle A970 centre (-328, 128) radius 1.85
  circle A971 centre (-336, 136) radius 1.85
  circle A972 centre (-344, 128) radius 1.85
  circle A973 centre (-336, 120) radius 1.85
  circle A974 centre (-328, 112) radius 1.85
  circle A975 centre (-336, 120) radius 1.85
  circle A976 centre (-344, 112) radius 1.85
  circle A977 centre (-336, 104) radius 1.85
  circle A978 centre (-328, 96) radius 1.85
  circle A979 centre (-336, 104) radius 1.85
  circle A980 centre (-344, 96) radius 1.85
  circle A981 centre (-336, 88) radius 1.85
  circle A982 centre (-328, 80) radius 1.85
  circle A983 centre (-336, 88) radius 1.85
  circle A984 centre (-344, 80) radius 1.85
  circle A985 centre (-336, 72) radius 1.85
  circle A986 centre (-328, 64) radius 1.85
  circle A987 centre (-336, 72) radius 1.85
  circle A988 centre (-344, 64) radius 1.85
  circle A989 centre (-336, 56) radius 1.85
  circle A990 centre (-328, 48) radius 1.85
  circle A991 centre (-336, 56) radius 1.85
  circle A992 centre (-344, 48) radius 1.85
  circle A993 centre (-336, 40) radius 1.85
  circle A994 centre (-328, 32) radius 1.85
  circle A995 centre (-336, 40) radius 1.85
  circle A996 centre (-344, 32) radius 1.85
  circle A997 centre (-336, 24) radius 1.85
  circle A998 centre (-328, 16) radius 1.85
  circle A999 centre (-336, 24) radius 1.85
  circle A1000 centre (-344, 16) radius 1.85
  circle A1001 centre (-336, 8) radius 1.85
  circle A1002 centre (-328, 0) radius 1.85
  circle A1003 centre (-336, 8) radius 1.85
  circle A1004 centre (-344, 0) radius 1.85
  circle A1005 centre (-336, -8) radius 1.85
  circle A1006 centre (-328, -16) radius 1.85
  circle A1007 centre (-336, -8) radius 1.85
  circle A1008 centre (-344, -16) radius 1.85
  circle A1009 centre (-336, -24) radius 1.85
  circle A1010 centre (-328, -32) radius 1.85
  circle A1011 centre (-336, -24) radius 1.85
  circle A1012 centre (-344, -32) radius 1.85
  circle A1013 centre (-336, -40) radius 1.85
  circle A1014 centre (-344, 128) radius 1.85
  circle A1015 centre (-352, 136) radius 1.85
  circle A1016 centre (-360, 128) radius 1.85
  circle A1017 centre (-352, 120) radius 1.85
  circle A1018 centre (-344, 112) radius 1.85
  circle A1019 centre (-352, 120) radius 1.85
  circle A1020 centre (-360, 112) radius 1.85
  circle A1021 centre (-352, 104) radius 1.85
  circle A1022 centre (-344, 96) radius 1.85
  circle A1023 centre (-352, 104) radius 1.85
  circle A1024 centre (-360, 96) radius 1.85
  circle A1025 centre (-352, 88) radius 1.85
  circle A1026 centre (-344, 80) radius 1.85
  circle A1027 centre (-352, 88) radius 1.85
  circle A1028 centre (-360, 80) radius 1.85
  circle A1029 centre (-352, 72) radius 1.85
  circle A1030 centre (-344, 64) radius 1.85
  circle A1031 centre (-352, 72) radius 1.85
  circle A1032 centre (-360, 64) radius 1.85
  circle A1033 centre (-352, 56) radius 1.85
  circle A1034 centre (-344, 48) radius 1.85
  circle A1035 centre (-352, 56) radius 1.85
  circle A1036 centre (-360, 48) radius 1.85
  circle A1037 centre (-352, 40) radius 1.85
  circle A1038 centre (-344, 32) radius 1.85
  circle A1039 centre (-352, 40) radius 1.85
  circle A1040 centre (-360, 32) radius 1.85
  circle A1041 centre (-352, 24) radius 1.85
  circle A1042 centre (-344, 16) radius 1.85
  circle A1043 centre (-352, 24) radius 1.85
  circle A1044 centre (-360, 16) radius 1.85
  circle A1045 centre (-352, 8) radius 1.85
  circle A1046 centre (-344, 0) radius 1.85
  circle A1047 centre (-352, 8) radius 1.85
  circle A1048 centre (-360, 0) radius 1.85
  circle A1049 centre (-352, -8) radius 1.85
  circle A1050 centre (-344, -16) radius 1.85
  circle A1051 centre (-352, -8) radius 1.85
  circle A1052 centre (-360, -16) radius 1.85
  circle A1053 centre (-352, -24) radius 1.85
  circle A1054 centre (-344, -32) radius 1.85
  circle A1055 centre (-352, -24) radius 1.85
  circle A1056 centre (-360, -32) radius 1.85
  circle A1057 centre (-352, -40) radius 1.85
  circle A1058 centre (-360, 128) radius 1.85
  circle A1059 centre (-368, 136) radius 1.85
  circle A1060 centre (-376, 128) radius 1.85
  circle A1061 centre (-368, 120) radius 1.85
  circle A1062 centre (-360, 112) radius 1.85
  circle A1063 centre (-368, 120) radius 1.85
  circle A1064 centre (-376, 112) radius 1.85
  circle A1065 centre (-368, 104) radius 1.85
  circle A1066 centre (-360, 96) radius 1.85
  circle A1067 centre (-368, 104) radius 1.85
  circle A1068 centre (-376, 96) radius 1.85
  circle A1069 centre (-368, 88) radius 1.85
  circle A1070 centre (-360, 80) radius 1.85
  circle A1071 centre (-368, 88) radius 1.85
  circle A1072 centre (-376, 80) radius 1.85
  circle A1073 centre (-368, 72) radius 1.85
  circle A1074 centre (-360, 64) radius 1.85
  circle A1075 centre (-368, 72) radius 1.85
  circle A1076 centre (-376, 64) radius 1.85
  circle A1077 centre (-368, 56) radius 1.85
  circle A1078 centre (-360, 48) radius 1.85
  circle A1079 centre (-368, 56) radius 1.85
  circle A1080 centre (-376, 48) radius 1.85
  circle A1081 centre (-368, 40) radius 1.85
  circle A1082 centre (-360, 32) radius 1.85
  circle A1083 centre (-368, 40) radius 1.85
  circle A1084 centre (-376, 32) radius 1.85
  circle A1085 centre (-368, 24) radius 1.85
  circle A1086 centre (-360, 16) radius 1.85
  circle A1087 centre (-368, 24) radius 1.85
  circle A1088 centre (-376, 16) radius 1.85
  circle A1089 centre (-368, 8) radius 1.85
  circle A1090 centre (-360, 0) radius 1.85
  circle A1091 centre (-368, 8) radius 1.85
  circle A1092 centre (-376, 0) radius 1.85
  circle A1093 centre (-368, -8) radius 1.85
  circle A1094 centre (-360, -16) radius 1.85
  circle A1095 centre (-368, -8) radius 1.85
  circle A1096 centre (-376, -16) radius 1.85
  circle A1097 centre (-368, -24) radius 1.85
  circle A1098 centre (-360, -32) radius 1.85
  circle A1099 centre (-368, -24) radius 1.85
  circle A1100 centre (-376, -32) radius 1.85
  circle A1101 centre (-368, -40) radius 1.85
  point P0 (0, 0)
  dimension "d0" = 416
  dimension "d1" = 192
  dimension "d4" = 16
  dimension "d7" = 16
  constraints: 1102 centre point, 8 end point, 2 horizontal, 2 parallel, 1 perpendicular, 1 vertical, 2205 other
  measures "d0" distance of L2.end L1.end
  measures "d1" distance of L1.end L0.end
  measures "d4" distance of A0.centre A6.centre
  measures "d7" distance of A0.centre A46.centre
extrude "Extrusion1" add sketch "Sketch2" along normal blind 2